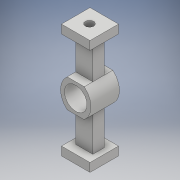
# Autodesk Inventor part: PuenteMandibula
Saved by Autodesk Inventor 2017 SP1 (Build 210196100, 196)
## iProperties
Part Number: PuenteMandibula
Material: Genérico
Document SubType Name: Modeling
Designer: Juan
Density: 1 g/cm^3
Appearance: Valor por defecto
Author: Juan
Autodesk Inventor part; units mm, degrees
sketch "Boceto1" plane through (0, 0, 0) normal (0, 1, 0) x (-1, 0, 0)
  line L0 (0, 40) -> (10, 40)
  line L1 (10, 40) -> (10, 37)
  line L2 (10, 37) -> (8, 37)
  line L3 (8, 37) -> (8, 25)
  arc A0 (8, 15) -> (8, 25) centre (3.8467, 20) ccw
  line L4 (8, 15) -> (8, 3)
  line L5 (8, 3) -> (10, 3)
  line L6 (10, 3) -> (10, 0)
  line L7 (10, 0) -> (0, 0)
  line L8 (0, 40) -> (0, 37)
  line L9 (0, 37) -> (2, 37)
  line L10 (2, 37) -> (2, 25)
  arc A1 (2, 25) -> (2, 15) centre (6.1533, 20) ccw
  line L11 (2, 15) -> (2, 3)
  line L12 (2, 3) -> (0, 3)
  line L13 (0, 3) -> (0, 0)
  dimension "d0" = 10
  dimension "d1" = 3
  dimension "d2" = 2
  dimension "d3" = 12
  dimension "d4" = 10
  dimension "d5" = 6.5
  dimension "d6" = 12
  dimension "d7" = 3
  dimension "d8" = 10
  dimension "d9" = 2
  dimension "d10" = 10
  dimension "d19" = 6.5
  dimension "d44" = 12
  dimension "d45" = 12
  constraints: 28 end point, 10 perpendicular, 4 point on circle, 3 vertical, 2 centre point, 1 coincident, 1 horizontal
  measures "d0" distance of L0.start L0.end
  measures "d1" distance of L0.end L1.end
  measures "d2" distance of L1.end L2.end
  measures "d3" distance of L2.end L3.end
  measures "d4" distance of L3.end L4.start
  measures "d5" radius of A0
  measures "d6" distance of L4.start L4.end
  measures "d7" distance of L5.end L6.end
  measures "d8" distance of L6.end L7.end
  measures "d9" distance of L8.end L9.end
  measures "d10" distance of L10.end L11.start
  measures "d19" radius of A1
  measures "d44" distance of L11.start L11.end
  measures "d45" distance of L9.end L10.end
extrude "Extrusión1" add sketch "Boceto1" along normal blind 10
ref_plane "Plano de trabajo1" through (0, 10, 0) normal (0, 1, 0) x (1, 0, 0)
sketch "Boceto2" plane through (0, 10, 0) normal (0, 1, 0) x (1, 0, 0)
  line L0 (-8, -37) -> (-8, -25) projected
  arc A0 (-2, -25) -> (-2, -15) centre (-6.1533, -20) ccw projected
  line L1 (-8, -37) -> (-2, -37)
  line L2 (-2, -37) -> (-2, -25)
  line L3 (-2, -25) -> (-8, -25)
  line L4 (-8, -25) -> (-8, -37)
  line L5 (-8, -3) -> (-8, -15) projected
  line L6 (-2, -15) -> (-2, -3) projected
  line L7 (-8, -15) -> (-2, -15)
  line L8 (-2, -15) -> (-2, -3)
  line L9 (-2, -3) -> (-8, -3)
  line L10 (-8, -3) -> (-8, -15)
  point P0 (0, 0)
  constraints: 16 end point, 4 parallel, 2 horizontal, 2 perpendicular
extrude "Extrusión2" cut sketch "Boceto2" against normal blind 3
ref_plane "Plano de trabajo2" through (0, 0, 0) normal (0, -1, 0) x (1, 0, 0)
sketch "Boceto3" plane through (0, 0, 0) normal (0, -1, 0) x (1, 0, 0)
  line L0 (-2, 25) -> (-2, 37) projected
  line L1 (-8, 25) -> (-2, 25) projected
  line L2 (-2, 37) -> (-8, 37)
  line L3 (-8, 37) -> (-8, 25)
  line L4 (-8, 25) -> (-2, 25)
  line L5 (-2, 25) -> (-2, 37)
  arc A0 (-2, 15) -> (-2, 25) centre (-6.1533, 20) ccw projected
  line L6 (-8, 3) -> (-10, 3) projected
  line L7 (-2, 15) -> (-8, 15)
  line L8 (-8, 15) -> (-8, 3)
  line L9 (-8, 3) -> (-2, 3)
  line L10 (-2, 3) -> (-2, 15)
  point P0 (0, 0)
  constraints: 16 end point, 4 parallel, 2 horizontal, 2 perpendicular
extrude "Extrusión3" cut sketch "Boceto3" against normal blind 3
ref_plane "Plano de trabajo3" through (0, 10, 0) normal (0, 1, 0) x (1, 0, 0)
sketch "Boceto4" plane through (0, 10, 0) normal (0, 1, 0) x (1, 0, 0)
  line L0 (-2, -25) -> (-8, -25) construction
  line L1 (-8, -15) -> (-2, -25) construction
  arc A0 (-8, -15) -> (-8, -25) centre (-3.8467, -20) ccw construction
  line L2 (-2, -15) -> (-8, -25) construction
  line L3 (-5, -20) -> (0.3148, -20) construction
  point P0 (0, 0)
  constraints: 6 end point, 1 horizontal, 1 midpoint
hole "Agujero1" at (-5, 10, 20) direction (0, -1, 0) diameter 8 end through all
ref_plane "Plano de trabajo4" through (0, 0, 0) normal (0, 0, -1) x (-1, 0, 0)
sketch "Boceto5" plane through (0, 0, 0) normal (0, 0, -1) x (-1, 0, 0)
  line L0 (10, 10) -> (0, 0) construction
  line L1 (0, 0) -> (0, 10) construction
  line L2 (10, 0) -> (10, 10) construction
  line L3 (0, 10) -> (10, 0) construction
  line L4 (5, 5) -> (5, 10) construction
  line L5 (0, 10) -> (10, 10) construction
  constraints: 6 end point, 2 midpoint
hole "Agujero2" at (-5, 5, 0) direction (0, 0, 1) diameter 3 depth 3 tip angle 118
ref_plane "Plano de trabajo5" through (-10, 0, 40) normal (0, 0, 1) x (1, 0, 0)
sketch "Boceto6" plane through (-10, 0, 40) normal (0, 0, 1) x (1, 0, 0)
  line L0 (10, 0) -> (10, 10) construction
  line L1 (-0.3467, 0) -> (2, 0) construction
  line L2 (10, 10) -> (-0.3467, 0) construction
  line L3 (2, 10) -> (-0.3467, 10) construction
  line L4 (-0.3467, 10) -> (10, 0) construction
  line L5 (4.8267, 5) -> (4.8267, 10) construction
  line L6 (0, 10) -> (10, 10) construction
  constraints: 6 end point, 1 midpoint, 1 point on line, 1 vertical
hole "Agujero3" at (-5.1733, 5, 40) direction (0, 0, -1) diameter 3 depth 3 tip angle 118
equation "\"d3\" = d6"
equation "\"d44\" = d6"
equation "\"d45\" = d6"
